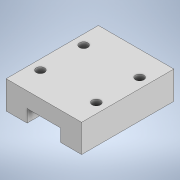
# Autodesk Inventor part: slider_move
Saved by Autodesk Inventor 2022 (Build 260153070, 153G)
## iProperties
Created: 2022-08-15
Part Number: slider_move
Material: 一般
Document SubType Name: Modeling
Designer: zegi
Density: 1 g/cm^3
Appearance: 既定
Author: zegi
Autodesk Inventor part; units mm, degrees
ref_plane "YZ Plane" through (0, 0, 0) normal (1, 0, 0) x (0, 1, 0)
ref_plane "XZ Plane" through (0, 0, 0) normal (0, 1, 0) x (-1, 0, 0)
ref_plane "XY Plane" through (0, 0, 0) normal (0, 0, 1) x (1, 0, 0)
sketch "スケッチ1" plane through (0, 0, 0) normal (0, 0, 1) x (1, 0, 0)
  line L0 (0, 0) -> (12, 0)
  line L1 (12, 0) -> (12, 7.5)
  line L2 (12, 7.5) -> (0, 7.5)
  line L3 (0, 7.5) -> (0, 0)
  line L4 (-7.5, 13) -> (19.5, 13)
  line L5 (-7.5, 13) -> (-7.5, 3)
  line L6 (19.5, 13) -> (19.5, 3)
  line L7 (-7.5, 3) -> (0, 3)
  line L8 (12, 3) -> (19.5, 3)
  dimension "d0" = 12
  dimension "d1" = 7.5
  dimension "d2" = 13
  dimension "d3" = 10
  dimension "d4" = 10
  dimension "d5" = 27
  dimension "d6" = 7.5
  constraints: 18 end point, 3 point on line, 2 horizontal, 2 parallel, 2 perpendicular, 2 vertical
  measures "d0" distance of L2.end L1.end
  measures "d1" distance of L1.end L0.end
  measures "d2" distance between parallel lines of L0 L4
  measures "d3" distance of L4.start L5.end
  measures "d4" distance of L4.end L6.end
  measures "d5" distance of L4.start L4.end
  measures "d6" distance between parallel lines of L6 L1
extrude "押し出し1" add sketch "スケッチ1" along normal blind 33 contours L7 L5 L4 L6 L8 L1 L2 L3
sketch "スケッチ2" plane through (-7.5, 13, 0) normal (0, 1, 0) x (1, 0, 0)
  line L0 (0, 0) -> (7.5, 0) projected
  line L1 (0, -33) -> (7.5, -33) projected
  line L2 (7.5, 0) -> (19.5, 0) projected
  line L3 (3.5, 0) -> (3.5, -33)
  line L4 (23.5, 0) -> (23.5, -33)
  line L5 (0, 0) -> (0, -33) projected
  line L6 (27, 0) -> (27, -33) projected
  point P0 (3.5, -24.25)
  point P1 (3.5, -8.75)
  point P2 (23.5, -24.25)
  point P3 (23.5, -8.75)
  dimension "d9" = 3.5
  dimension "d10" = 3.5
  dimension "d11" = 15.5
  dimension "d12" = 8.75
  dimension "d13" = 33
  constraints: 6 point on line, 4 end point, 2 vertical
  measures "d9" distance between parallel lines of L5 L3
  measures "d10" distance between parallel lines of L6 L4
  measures "d11" distance of point (3.5, -8.75) point (3.5, -24.25)
  measures "d12" distance from line of point (3.5, -8.75) L0
  measures "d13" distance of L0.start L1.start
hole "穴1" at (-4, 13, 24.25) at (-4, 13, 8.75) at (16, 13, 24.25) at (16, 13, 8.75) direction (0, -1, 0) diameter 3 depth 3 tip angle 118
equation "\"d6\" = -0.5 * d0 + 0.5 * d5"
equation "\"d12\" = -0.5 * d11 + 0.5 * d13"
